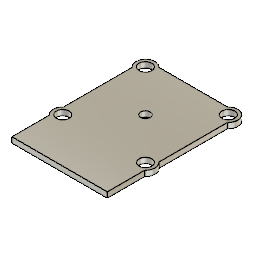
_Piezo Sensor Mock.27c4ffc2-d7b1-423b-bce0-f19f87cd386d (Autodesk Fusion 360 design; units mm, degrees)
Autodesk Fusion 360 part; units mm, degrees
sketch "Sketch1" plane through (0, 0, 0) normal (0, 0, 1) x (1, 0, 0)
  line L0 (0, 0) -> (30, 0)
  line L1 (30, 0) -> (30, 42)
  line L2 (30, 42) -> (0, 42)
  line L3 (0, 42) -> (0, 0)
  circle A0 centre (2, 40) radius 2
  circle A1 centre (28, 40) radius 2
  circle A2 centre (2, 14) radius 2
  circle A3 centre (28, 14) radius 2
  circle A4 centre (2, 40) radius 3
  circle A5 centre (28, 40) radius 3
  circle A6 centre (28, 14) radius 3
  circle A7 centre (2, 14) radius 3
  circle A8 centre (15, 27) radius 1.5
  dimension "d1" = 30
  dimension "d2" = 42
  dimension "d3" = 4
  dimension "d6" = 26
  dimension "d7" = -26
  dimension "d8" = 6
  dimension "d9" = 6
  dimension "d10" = 6
  dimension "d11" = 6
  dimension "d14" = 3
  dimension "d15" = 15
  dimension "d16" = 15
  constraint horizontal L0
  constraint vertical L1
  constraint horizontal L2
  constraint vertical L3
  constraint coincident L0.start L3.end
  constraint concentric A0 A4
  constraint concentric A1 A5
  constraint concentric A3 A6
  constraint concentric A2 A7
  measures "d1" distance of L0.start L0.end
  measures "d2" distance of L0.start L2.end
  measures "d3" diameter of A0
  measures "d8" diameter of A4
  measures "d9" diameter of A5
  measures "d10" diameter of A6
  measures "d11" diameter of A7
  measures "d14" diameter of A8
  measures "d15" distance of L2 A8.centre
  measures "d16" distance of L1 A8.centre
extrude "Extrude1" add sketch "Sketch1" along normal blind 1.75 contours L0 L1 L2 L3 A4 A5 A6 A7 | L3 A7 | L3 A7 | L1 A6 | L1 A6 | L2 L3 A4 | L2 L3 A0 A4 | L1 L2 A1 A5 | L1 L2 A5 | L2 L3 A0 | L1 L2 A1
